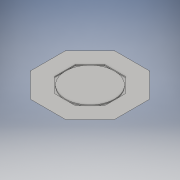
# Autodesk Inventor part: Case
Saved by Autodesk Inventor 2016 SP2 (Build 200236200, 236)
## iProperties
Created: 2018-06-28
Part Number: Case
Material: Generisch
Document SubType Name: Modeling
Designer: Nils
Density: 1 g/cm^3
Appearance: Vorgabe
Author: Nils
Autodesk Inventor part; units mm, degrees
ref_plane "YZ Plane" through (0, 0, 0) normal (1, 0, 0) x (0, 1, 0)
ref_plane "XZ Plane" through (0, 0, 0) normal (0, 1, 0) x (-1, 0, 0)
ref_plane "XY Plane" through (0, 0, 0) normal (0, 0, 1) x (1, 0, 0)
sketch "Skizze1" plane through (0, 0, 0) normal (0, 0, 1) x (1, 0, 0)
  line L0 (60.3553, 25) -> (60.3553, -25)
  line L1 (60.3553, -25) -> (25, -60.3553)
  line L2 (25, -60.3553) -> (-25, -60.3553)
  line L3 (-25, -60.3553) -> (-60.3553, -25)
  line L4 (-60.3553, -25) -> (-60.3553, 25)
  line L5 (-60.3553, 25) -> (-25, 60.3553)
  line L6 (-25, 60.3553) -> (25, 60.3553)
  line L7 (25, 60.3553) -> (60.3553, 25)
  line L8 (-25, -60.3553) -> (25, 60.3553) construction
  circle A0 centre (0, 0) radius 50
  dimension "d10" = 50
  dimension "d11" = 100
  constraints: 18 end point, 2 coincident, 1 centre point, 1 vertical, 17 other
  measures "d10" distance of L0.start L0.end
  measures "d11" diameter of A0
sketch "Skizze3" plane through (0, 0, 0) normal (0, 1, 0) x (-1, 0, 0)
  circle A0 centre (-60.3553, 8.75) radius 5.25
  line L0 (-51.6053, 0) -> (-51.6053, 17.5)
  line L1 (-51.6053, 17.5) -> (-86.2536, 17.5)
  line L2 (-51.6053, 0) -> (-60.3553, 0)
  line L3 (-60.3553, 0) -> (-86.2536, 17.5)
  point P0 (0, 0)
  point P1 (-60.3553, 0)
  dimension "d4" = 10.5
  dimension "d12" = 8.75
  dimension "d13" = 8.75
  dimension "d14" = 7.25
  dimension "d16" = 0
  dimension "d21" = 8.75
  constraints: 8 end point, 1 centre point, 1 horizontal, 1 perpendicular, 1 vertical
  measures "d4" diameter of A0
  measures "d12" distance from line of L1 A0.centre
  measures "d13" distance of point (-60.355, 0) A0.centre
  measures "d14" distance from line of L3 A0.centre
  measures "d16" horizontal distance of point (-60.355, 0) A0.centre
  measures "d21" distance of point (-60.355, 0) L0.start
sweep "Sweeping2" add profiles "Skizze3" path "Skizze1" path curves L0 L7 L6 L5 L4 L3 L2 L1
sketch "Skizze4" plane through (25, -60.3553, 0) normal (0, 0, -1) x (-1, 0, 0)
  circle A0 centre (25, 60.3553) radius 50
  line L0 (-35.3553, 35.3553) -> (-35.3553, 85.3553) projected
  line L1 (0, 0) -> (-35.3553, 35.3553) projected
  line L2 (50, 0) -> (0, 0) projected
  line L3 (85.3553, 35.3553) -> (50, 0) projected
  line L4 (85.3553, 85.3553) -> (85.3553, 35.3553) projected
  line L5 (50, 120.7107) -> (85.3553, 85.3553) projected
  line L6 (0, 120.7107) -> (50, 120.7107) projected
  line L7 (-35.3553, 85.3553) -> (0, 120.7107) projected
  line L8 (-26.6053, 81.731) -> (3.6244, 111.9607) projected
  line L9 (3.6244, 111.9607) -> (46.3756, 111.9607) projected
  line L10 (46.3756, 111.9607) -> (76.6053, 81.731) projected
  line L11 (76.6053, 81.731) -> (76.6053, 38.9797) projected
  line L12 (76.6053, 38.9797) -> (46.3756, 8.75) projected
  line L13 (46.3756, 8.75) -> (3.6244, 8.75) projected
  line L14 (3.6244, 8.75) -> (-26.6053, 38.9797) projected
  line L15 (-26.6053, 38.9797) -> (-26.6053, 81.731) projected
  dimension "d22" = 100
  constraints: 1 centre point, 1 coincident
  measures "d22" diameter of A0
extrude "Extrusion1" add sketch "Skizze4" against normal blind 15.5 contours L8 L9 L10 L11 L12 L13 L14 L15
sketch "Skizze5" plane through (-35.7274, 86.2536, 17.5) normal (0, 0, 1) x (1, 0, 0)
  circle A0 centre (35.7274, -86.2536) radius 50 projected
extrude "Extrusion2" add sketch "Skizze5" against normal blind 5
sketch "Skizze7" plane through (0, 0, 12.5) normal (0, 0, -1) x (-1, 0, 0)
  line L0 (7, 5.5) -> (-7, 5.5)
  line L1 (-7, 5.5) -> (-7, -5.5)
  line L2 (-7, -5.5) -> (7, -5.5)
  line L3 (7, -5.5) -> (7, 5.5)
  line L4 (7, 5.5) -> (-7, -5.5) construction
  line L5 (-7, 5.5) -> (7, -5.5) construction
  line L6 (7, -11.5) -> (-7, -11.5)
  line L7 (-7, -11.5) -> (-7, -22.5)
  line L8 (-7, -22.5) -> (7, -22.5)
  line L9 (7, -22.5) -> (7, -11.5)
  line L10 (7, -11.5) -> (-7, -22.5) construction
  line L11 (-7, -11.5) -> (7, -22.5) construction
  line L12 (13.1003, 3.1037) -> (8.774, -10.2111)
  line L13 (8.774, -10.2111) -> (19.2357, -13.6103)
  line L14 (19.2357, -13.6103) -> (23.5619, -0.2955)
  line L15 (23.5619, -0.2955) -> (13.1003, 3.1037)
  line L16 (13.1003, 3.1037) -> (19.2357, -13.6103) construction
  line L17 (8.774, -10.2111) -> (23.5619, -0.2955) construction
  line L18 (1.0964, 13.4182) -> (12.4226, 5.1892)
  line L19 (12.4226, 5.1892) -> (18.8883, 14.0884)
  line L20 (18.8883, 14.0884) -> (7.562, 22.3174)
  line L21 (7.562, 22.3174) -> (1.0964, 13.4182)
  line L22 (1.0964, 13.4182) -> (18.8883, 14.0884) construction
  line L23 (12.4226, 5.1892) -> (7.562, 22.3174) construction
  line L24 (-12.4226, 5.1892) -> (-1.0964, 13.4182)
  line L25 (-1.0964, 13.4182) -> (-7.562, 22.3174)
  line L26 (-7.562, 22.3174) -> (-18.8883, 14.0884)
  line L27 (-18.8883, 14.0884) -> (-12.4226, 5.1892)
  line L28 (-12.4226, 5.1892) -> (-7.562, 22.3174) construction
  line L29 (-1.0964, 13.4182) -> (-18.8883, 14.0884) construction
  line L30 (-8.774, -10.2111) -> (-13.1003, 3.1037)
  line L31 (-13.1003, 3.1037) -> (-23.5619, -0.2955)
  line L32 (-23.5619, -0.2955) -> (-19.2357, -13.6103)
  line L33 (-19.2357, -13.6103) -> (-8.774, -10.2111)
  line L34 (-8.774, -10.2111) -> (-23.5619, -0.2955) construction
  line L35 (-13.1003, 3.1037) -> (-19.2357, -13.6103) construction
  line L36 (0, 0) -> (0, -50) construction
  line L37 (7, -27.5) -> (-7, -27.5)
  line L38 (-7, -27.5) -> (-7, -38.5)
  line L39 (-7, -38.5) -> (7, -38.5)
  line L40 (7, -38.5) -> (7, -27.5)
  line L41 (7, -27.5) -> (-7, -38.5) construction
  line L42 (-7, -27.5) -> (7, -38.5) construction
  line L43 (19.8122, -20.3157) -> (7.6878, -27.3157)
  line L44 (7.6878, -27.3157) -> (25.3122, -29.842) construction
  line L45 (19.8122, -20.3157) -> (13.1878, -36.842) construction
  line L46 (13.1878, -36.842) -> (25.3122, -29.842)
  line L47 (7.6878, -27.3157) -> (13.1878, -36.842)
  line L48 (25.3122, -29.842) -> (19.8122, -20.3157)
  line L49 (27.3157, -7.6878) -> (20.3157, -19.8122)
  line L50 (20.3157, -19.8122) -> (36.842, -13.1878) construction
  line L51 (27.3157, -7.6878) -> (29.842, -25.3122) construction
  line L52 (29.842, -25.3122) -> (36.842, -13.1878)
  line L53 (20.3157, -19.8122) -> (29.842, -25.3122)
  line L54 (36.842, -13.1878) -> (27.3157, -7.6878)
  line L55 (27.5, 7) -> (27.5, -7)
  line L56 (27.5, -7) -> (38.5, 7) construction
  line L57 (27.5, 7) -> (38.5, -7) construction
  line L58 (38.5, -7) -> (38.5, 7)
  line L59 (27.5, -7) -> (38.5, -7)
  line L60 (38.5, 7) -> (27.5, 7)
  line L61 (20.3157, 19.8122) -> (27.3157, 7.6878)
  line L62 (27.3157, 7.6878) -> (29.842, 25.3122) construction
  line L63 (20.3157, 19.8122) -> (36.842, 13.1878) construction
  line L64 (36.842, 13.1878) -> (29.842, 25.3122)
  line L65 (27.3157, 7.6878) -> (36.842, 13.1878)
  line L66 (29.842, 25.3122) -> (20.3157, 19.8122)
  line L67 (7.6878, 27.3157) -> (19.8122, 20.3157)
  line L68 (19.8122, 20.3157) -> (13.1878, 36.842) construction
  line L69 (7.6878, 27.3157) -> (25.3122, 29.842) construction
  line L70 (25.3122, 29.842) -> (13.1878, 36.842)
  line L71 (19.8122, 20.3157) -> (25.3122, 29.842)
  line L72 (13.1878, 36.842) -> (7.6878, 27.3157)
  line L73 (-7, 27.5) -> (7, 27.5)
  line L74 (7, 27.5) -> (-7, 38.5) construction
  line L75 (-7, 27.5) -> (7, 38.5) construction
  line L76 (7, 38.5) -> (-7, 38.5)
  line L77 (7, 27.5) -> (7, 38.5)
  line L78 (-7, 38.5) -> (-7, 27.5)
  line L79 (-19.8122, 20.3157) -> (-7.6878, 27.3157)
  line L80 (-7.6878, 27.3157) -> (-25.3122, 29.842) construction
  line L81 (-19.8122, 20.3157) -> (-13.1878, 36.842) construction
  line L82 (-13.1878, 36.842) -> (-25.3122, 29.842)
  line L83 (-7.6878, 27.3157) -> (-13.1878, 36.842)
  line L84 (-25.3122, 29.842) -> (-19.8122, 20.3157)
  line L85 (-27.3157, 7.6878) -> (-20.3157, 19.8122)
  line L86 (-20.3157, 19.8122) -> (-36.842, 13.1878) construction
  line L87 (-27.3157, 7.6878) -> (-29.842, 25.3122) construction
  line L88 (-29.842, 25.3122) -> (-36.842, 13.1878)
  line L89 (-20.3157, 19.8122) -> (-29.842, 25.3122)
  line L90 (-36.842, 13.1878) -> (-27.3157, 7.6878)
  line L91 (-27.5, -7) -> (-27.5, 7)
  line L92 (-27.5, 7) -> (-38.5, -7) construction
  line L93 (-27.5, -7) -> (-38.5, 7) construction
  line L94 (-38.5, 7) -> (-38.5, -7)
  line L95 (-27.5, 7) -> (-38.5, 7)
  line L96 (-38.5, -7) -> (-27.5, -7)
  line L97 (-20.3157, -19.8122) -> (-27.3157, -7.6878)
  line L98 (-27.3157, -7.6878) -> (-29.842, -25.3122) construction
  line L99 (-20.3157, -19.8122) -> (-36.842, -13.1878) construction
  line L100 (-36.842, -13.1878) -> (-29.842, -25.3122)
  line L101 (-27.3157, -7.6878) -> (-36.842, -13.1878)
  line L102 (-29.842, -25.3122) -> (-20.3157, -19.8122)
  line L103 (-7.6878, -27.3157) -> (-19.8122, -20.3157)
  line L104 (-19.8122, -20.3157) -> (-13.1878, -36.842) construction
  line L105 (-7.6878, -27.3157) -> (-25.3122, -29.842) construction
  line L106 (-25.3122, -29.842) -> (-13.1878, -36.842)
  line L107 (-19.8122, -20.3157) -> (-25.3122, -29.842)
  line L108 (-13.1878, -36.842) -> (-7.6878, -27.3157)
  point P0 (0, -17)
  point P1 (16.168, -5.2533)
  point P2 (9.9923, 13.7533)
  point P3 (-9.9923, 13.7533)
  point P4 (-16.168, -5.2533)
  point P5 (0, -33)
  point P6 (16.5, -28.5788)
  point P7 (28.5788, -16.5)
  point P8 (33, 0)
  point P9 (28.5788, 16.5)
  point P10 (16.5, 28.5788)
  point P11 (0, 33)
  point P12 (-16.5, 28.5788)
  point P13 (-28.5788, 16.5)
  point P14 (-33, 0)
  point P15 (-28.5788, -16.5)
  point P16 (-16.5, -28.5788)
  dimension "d27" = 14
  dimension "d28" = 11
  dimension "d29" = 14
  dimension "d30" = 11
  dimension "d31" = 6
  dimension "d34" = 360
  dimension "d36" = 14
  dimension "d37" = 11
  dimension "d38" = 5
  dimension "d41" = 360
  constraints: 218 end point, 36 midpoint, 6 parallel, 3 horizontal, 3 perpendicular, 1 collinear, 1 point on line, 1 vertical, 189 other
  measures "d27" distance of L2.end L1.end
  measures "d28" distance of L1.end L0.end
  measures "d29" distance of L8.end L7.end
  measures "d30" distance of L7.end L6.end
  measures "d31" distance between parallel lines of L2 L6
  measures "d36" distance of L39.end L38.end
  measures "d37" distance of L38.end L37.end
  measures "d38" distance between parallel lines of L8 L37
extrude "Extrusion3" add sketch "Skizze7" along normal blind 3
equation "\"d13\" = d12"
equation "\"d21\" = d13"
